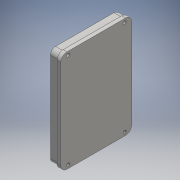
# Autodesk Inventor part: ET7
Saved by Autodesk Inventor 2016 (Build 200138000, 138)
## iProperties
Created: 2016-03-20
Part Number: ET7
Material: Genérico
Document SubType Name: Modeling
Designer: Usuario1
Density: 1 g/cm^3
Appearance: Valor por defecto
Author: Usuario1
Autodesk Inventor part; units mm, degrees
ref_plane "YZ Plane" through (0, 0, 0) normal (1, 0, 0) x (0, 1, 0)
ref_plane "XZ Plane" through (0, 0, 0) normal (0, 1, 0) x (-1, 0, 0)
ref_plane "XY Plane" through (0, 0, 0) normal (0, 0, 1) x (1, 0, 0)
sketch "Boceto1" plane through (0, 0, 0) normal (1, 0, 0) x (0, 1, 0)
  line L0 (2.3957, 0.3049) -> (2.3957, 0.0787)
  line L1 (2.3957, 0.0787) -> (2.2436, 0.0787)
  line L2 (2.2436, 0.0787) -> (2.2436, 0.3049)
  line L3 (2.2436, 0.3049) -> (2.3957, 0.3049)
  circle A0 centre (0.5248, 3.3826) radius 0.0547
  line L4 (0.5812, 3.113) -> (0.5812, 2.8452)
  line L5 (0.5812, 2.8452) -> (0.4683, 2.8452)
  line L6 (0.4683, 2.8452) -> (0.4683, 3.113)
  line L7 (0.4683, 3.113) -> (0.5812, 3.113)
  line L8 (0.5812, 2.5971) -> (0.5812, 2.3293)
  line L9 (0.5812, 2.3293) -> (0.4683, 2.3293)
  line L10 (0.4683, 2.3293) -> (0.4683, 2.5971)
  line L11 (0.4683, 2.5971) -> (0.5812, 2.5971)
  line L12 (0.5812, 2.0812) -> (0.5812, 1.8134)
  line L13 (0.5812, 1.8134) -> (0.4683, 1.8134)
  line L14 (0.4683, 1.8134) -> (0.4683, 2.0812)
  line L15 (0.4683, 2.0812) -> (0.5812, 2.0812)
  line L16 (0.5812, 1.5653) -> (0.5812, 1.2975)
  line L17 (0.5812, 1.2975) -> (0.4683, 1.2975)
  line L18 (0.4683, 1.2975) -> (0.4683, 1.5653)
  line L19 (0.4683, 1.5653) -> (0.5812, 1.5653)
  line L20 (0.5812, 1.0494) -> (0.5812, 0.7816)
  line L21 (0.5812, 0.7816) -> (0.4683, 0.7816)
  line L22 (0.4683, 0.7816) -> (0.4683, 1.0494)
  line L23 (0.4683, 1.0494) -> (0.5812, 1.0494)
  line L24 (1.2433, 0.3049) -> (1.2433, 0.0787)
  line L25 (1.2433, 0.0787) -> (1.0912, 0.0787)
  line L26 (1.0912, 0.0787) -> (1.0912, 0.3049)
  line L27 (1.0912, 0.3049) -> (1.2433, 0.3049)
  line L28 (0.5861, 0.3049) -> (0.5861, 0.0787)
  line L29 (0.5861, 0.0787) -> (0.434, 0.0787)
  line L30 (0.434, 0.0787) -> (0.434, 0.3049)
  line L31 (0.434, 0.3049) -> (0.5861, 0.3049)
  line L32 (2.7629, 3.0481) -> (2.7629, 2.6834)
  line L33 (2.7629, 2.6834) -> (2.9608, 2.6834)
  line L34 (2.9608, 2.6834) -> (2.9608, 3.0481)
  line L35 (2.9608, 3.0481) -> (2.7629, 3.0481)
  line L36 (2.7629, 2.4411) -> (2.7629, 1.0453)
  line L37 (2.7629, 1.0453) -> (2.817, 1.0453)
  line L38 (2.817, 1.0453) -> (2.817, 2.4411)
  line L39 (2.817, 2.4411) -> (2.7629, 2.4411)
  circle A1 centre (2.483, -0.1054) radius 0.0623
  circle A2 centre (0.2799, -0.1054) radius 0.0623
  circle A3 centre (0.2799, 3.5918) radius 0.0623
  line L40 (2.7629, 3.4863) -> (2.7629, 0)
  arc A4 (2.5229, -0.24) -> (2.7629, 0) centre (2.5229, 0) ccw
  line L41 (2.5229, -0.24) -> (0.24, -0.24)
  arc A5 (0, 0) -> (0.24, -0.24) centre (0.24, 0) ccw
  line L42 (0, 0) -> (0, 3.4863)
  arc A6 (0.24, 3.7263) -> (0, 3.4863) centre (0.24, 3.4863) ccw
  line L43 (0.24, 3.7263) -> (2.5229, 3.7263)
  arc A7 (2.7629, 3.4863) -> (2.5229, 3.7263) centre (2.5229, 3.4863) ccw
  line L44 (0.0443, 3.4821) -> (0.0443, 0.0043)
  arc A8 (0.0443, 0.0043) -> (0.2443, -0.1957) centre (0.2443, 0.0043) ccw
  line L45 (0.2443, -0.1957) -> (2.5186, -0.1957)
  arc A9 (2.5186, -0.1957) -> (2.7186, 0.0043) centre (2.5186, 0.0043) ccw
  line L46 (2.7186, 0.0043) -> (2.7186, 3.4821)
  arc A10 (2.7186, 3.4821) -> (2.5186, 3.6821) centre (2.5186, 3.4821) ccw
  line L47 (2.5186, 3.6821) -> (0.2443, 3.6821)
  arc A11 (0.2443, 3.6821) -> (0.0443, 3.4821) centre (0.2443, 3.4821) ccw
  circle A12 centre (2.483, 3.5918) radius 0.0623
  line L48 (2.5087, 3.3303) -> (2.5087, 0.538)
  arc A13 (2.3887, 0.418) -> (2.5087, 0.538) centre (2.3887, 0.538) ccw
  line L49 (2.3887, 0.418) -> (0.8107, 0.418)
  arc A14 (0.6907, 0.538) -> (0.8107, 0.418) centre (0.8107, 0.538) ccw
  line L50 (0.6907, 0.538) -> (0.6907, 3.3303)
  arc A15 (0.8107, 3.4503) -> (0.6907, 3.3303) centre (0.8107, 3.3303) ccw
  line L51 (0.8107, 3.4503) -> (2.3887, 3.4503)
  arc A16 (2.5087, 3.3303) -> (2.3887, 3.4503) centre (2.3887, 3.3303) ccw
  line L52 (2.4044, 3.2168) -> (2.4044, 0.6515)
  arc A17 (2.3144, 0.5615) -> (2.4044, 0.6515) centre (2.3144, 0.6515) ccw
  line L53 (2.3144, 0.5615) -> (0.9806, 0.5615)
  arc A18 (0.8906, 0.6515) -> (0.9806, 0.5615) centre (0.9806, 0.6515) ccw
  line L54 (0.8906, 0.6515) -> (0.8906, 3.2168)
  arc A19 (0.9806, 3.3068) -> (0.8906, 3.2168) centre (0.9806, 3.2168) ccw
  line L55 (0.9806, 3.3068) -> (2.3144, 3.3068)
  arc A20 (2.4044, 3.2168) -> (2.3144, 3.3068) centre (2.3144, 3.2168) ccw
  point P0 (0, 0)
  constraints: 112 end point, 32 point on circle, 21 centre point, 4 point on line
extrude "Extrusión1" add sketch "Boceto1" against normal blind 0.15 contours L0 L1 L2 L3 | A0 | L4 L5 L6 L7 | L8 L9 L10 L11 | L12 L13 L14 L15 | L16 L17 L18 L19 | L20 L21 L22 L23 | L24 L25 L26 L27 | L28 L29 L30 L31 | L32 L40 L36 A4 L41 A5 L42 A6 L43 A7 | A11 L47 A10 L46 A9 L45 A8 L44 | L48 A13 L49 A14 L50 A15 L51 A16 | L52 A17 L53 A18 L54 A19 L55 A20
sketch "Boceto2" plane through (-0.15, 0, 0) normal (-1, 0, 0) x (0, 0, 1)
  circle A0 centre (3.5918, 2.483) radius 0.0623 projected
  circle A1 centre (3.5918, 0.2799) radius 0.0623 projected
  circle A2 centre (-0.1054, 0.2799) radius 0.0623 projected
  circle A3 centre (-0.1054, 2.483) radius 0.0623 projected
  line L0 (3.1814, 2.3957) -> (3.4077, 2.3957)
  line L1 (3.4077, 2.3957) -> (3.4077, 2.2436)
  line L2 (3.4077, 2.2436) -> (3.1814, 2.2436)
  line L3 (3.1814, 2.2436) -> (3.1814, 2.3957)
  circle A4 centre (0.1037, 0.5248) radius 0.0547
  line L4 (0.3734, 0.5812) -> (0.6411, 0.5812)
  line L5 (0.6411, 0.5812) -> (0.6411, 0.4683)
  line L6 (0.6411, 0.4683) -> (0.3734, 0.4683)
  line L7 (0.3734, 0.4683) -> (0.3734, 0.5812)
  line L8 (0.8893, 0.5812) -> (1.157, 0.5812)
  line L9 (1.157, 0.5812) -> (1.157, 0.4683)
  line L10 (1.157, 0.4683) -> (0.8893, 0.4683)
  line L11 (0.8893, 0.4683) -> (0.8893, 0.5812)
  line L12 (1.4052, 0.5812) -> (1.6729, 0.5812)
  line L13 (1.6729, 0.5812) -> (1.6729, 0.4683)
  line L14 (1.6729, 0.4683) -> (1.4052, 0.4683)
  line L15 (1.4052, 0.4683) -> (1.4052, 0.5812)
  line L16 (1.921, 0.5812) -> (2.1888, 0.5812)
  line L17 (2.1888, 0.5812) -> (2.1888, 0.4683)
  line L18 (2.1888, 0.4683) -> (1.921, 0.4683)
  line L19 (1.921, 0.4683) -> (1.921, 0.5812)
  line L20 (2.4369, 0.5812) -> (2.7047, 0.5812)
  line L21 (2.7047, 0.5812) -> (2.7047, 0.4683)
  line L22 (2.7047, 0.4683) -> (2.4369, 0.4683)
  line L23 (2.4369, 0.4683) -> (2.4369, 0.5812)
  line L24 (3.1814, 1.2433) -> (3.4077, 1.2433)
  line L25 (3.4077, 1.2433) -> (3.4077, 1.0912)
  line L26 (3.4077, 1.0912) -> (3.1814, 1.0912)
  line L27 (3.1814, 1.0912) -> (3.1814, 1.2433)
  line L28 (3.1814, 0.5861) -> (3.4077, 0.5861)
  line L29 (3.4077, 0.5861) -> (3.4077, 0.434)
  line L30 (3.4077, 0.434) -> (3.1814, 0.434)
  line L31 (3.1814, 0.434) -> (3.1814, 0.5861)
  line L32 (0.4382, 2.7629) -> (0.803, 2.7629)
  line L33 (0.803, 2.7629) -> (0.803, 2.9608)
  line L34 (0.803, 2.9608) -> (0.4382, 2.9608)
  line L35 (0.4382, 2.9608) -> (0.4382, 2.7629)
  line L36 (1.0453, 2.7629) -> (2.4411, 2.7629)
  line L37 (2.4411, 2.7629) -> (2.4411, 2.817)
  line L38 (2.4411, 2.817) -> (1.0453, 2.817)
  line L39 (1.0453, 2.817) -> (1.0453, 2.7629)
  circle A5 centre (3.5918, 2.483) radius 0.0623
  circle A6 centre (3.5918, 0.2799) radius 0.0623
  circle A7 centre (-0.1054, 0.2799) radius 0.0623
  line L40 (0, 2.7629) -> (3.4863, 2.7629)
  arc A8 (3.7263, 2.5229) -> (3.4863, 2.7629) centre (3.4863, 2.5229) ccw
  line L41 (3.7263, 2.5229) -> (3.7263, 0.24)
  arc A9 (3.4863, 0) -> (3.7263, 0.24) centre (3.4863, 0.24) ccw
  line L42 (3.4863, 0) -> (0, 0)
  arc A10 (-0.24, 0.24) -> (0, 0) centre (0, 0.24) ccw
  line L43 (-0.24, 0.24) -> (-0.24, 2.5229)
  arc A11 (0, 2.7629) -> (-0.24, 2.5229) centre (0, 2.5229) ccw
  line L44 (0.0043, 0.0443) -> (3.4821, 0.0443)
  arc A12 (3.4821, 0.0443) -> (3.6821, 0.2443) centre (3.4821, 0.2443) ccw
  line L45 (3.6821, 0.2443) -> (3.6821, 2.5186)
  arc A13 (3.6821, 2.5186) -> (3.4821, 2.7186) centre (3.4821, 2.5186) ccw
  line L46 (3.4821, 2.7186) -> (0.0043, 2.7186)
  arc A14 (0.0043, 2.7186) -> (-0.1957, 2.5186) centre (0.0043, 2.5186) ccw
  line L47 (-0.1957, 2.5186) -> (-0.1957, 0.2443)
  arc A15 (-0.1957, 0.2443) -> (0.0043, 0.0443) centre (0.0043, 0.2443) ccw
  circle A16 centre (-0.1054, 2.483) radius 0.0623
  line L48 (0.1561, 2.5087) -> (2.9483, 2.5087)
  arc A17 (3.0683, 2.3887) -> (2.9483, 2.5087) centre (2.9483, 2.3887) ccw
  line L49 (3.0683, 2.3887) -> (3.0683, 0.8107)
  arc A18 (2.9483, 0.6907) -> (3.0683, 0.8107) centre (2.9483, 0.8107) ccw
  line L50 (2.9483, 0.6907) -> (0.1561, 0.6907)
  arc A19 (0.0361, 0.8107) -> (0.1561, 0.6907) centre (0.1561, 0.8107) ccw
  line L51 (0.0361, 0.8107) -> (0.0361, 2.3887)
  arc A20 (0.1561, 2.5087) -> (0.0361, 2.3887) centre (0.1561, 2.3887) ccw
  line L52 (0.2695, 2.4044) -> (2.8349, 2.4044)
  arc A21 (2.9249, 2.3144) -> (2.8349, 2.4044) centre (2.8349, 2.3144) ccw
  line L53 (2.9249, 2.3144) -> (2.9249, 0.9806)
  arc A22 (2.8349, 0.8906) -> (2.9249, 0.9806) centre (2.8349, 0.9806) ccw
  line L54 (2.8349, 0.8906) -> (0.2695, 0.8906)
  arc A23 (0.1795, 0.9806) -> (0.2695, 0.8906) centre (0.2695, 0.9806) ccw
  line L55 (0.1795, 0.9806) -> (0.1795, 2.3144)
  arc A24 (0.2695, 2.4044) -> (0.1795, 2.3144) centre (0.2695, 2.3144) ccw
  point P0 (0, 0)
  constraints: 112 end point, 32 point on circle, 21 centre point, 4 point on line
extrude "Extrusión2" add sketch "Boceto2" along normal blind 0.3 contours L0 L1 L2 L3 | A4 | L4 L5 L6 L7 | L8 L9 L10 L11 | L12 L13 L14 L15 | L16 L17 L18 L19 | L20 L21 L22 L23 | L24 L25 L26 L27 | L28 L29 L30 L31 | A15 L47 A14 L46 A13 L45 A12 L44 | L48 A17 L49 A18 L50 A19 L51 A20 | L52 A21 L53 A22 L54 A23 L55 A24
sketch "Boceto3" plane through (-0.45, 0, 0) normal (-1, 0, 0) x (0, 0, 1)
  circle A0 centre (-0.1054, 2.483) radius 0.0623 projected
  circle A1 centre (-0.1054, 0.2799) radius 0.0623 projected
  circle A2 centre (3.5918, 0.2799) radius 0.0623 projected
  circle A3 centre (3.5918, 2.483) radius 0.0623 projected
  line L0 (0.0043, 0.0443) -> (3.4821, 0.0443) projected
  arc A4 (3.4821, 0.0443) -> (3.6821, 0.2443) centre (3.4821, 0.2443) ccw projected
  line L1 (3.6821, 0.2443) -> (3.6821, 2.5186) projected
  arc A5 (3.6821, 2.5186) -> (3.4821, 2.7186) centre (3.4821, 2.5186) ccw projected
  line L2 (3.4821, 2.7186) -> (0.0043, 2.7186) projected
  arc A6 (0.0043, 2.7186) -> (-0.1957, 2.5186) centre (0.0043, 2.5186) ccw projected
  line L3 (-0.1957, 2.5186) -> (-0.1957, 0.2443) projected
  arc A7 (-0.1957, 0.2443) -> (0.0043, 0.0443) centre (0.0043, 0.2443) ccw projected
  line L4 (3.1814, 2.3957) -> (3.4077, 2.3957)
  line L5 (3.4077, 2.3957) -> (3.4077, 2.2436)
  line L6 (3.4077, 2.2436) -> (3.1814, 2.2436)
  line L7 (3.1814, 2.2436) -> (3.1814, 2.3957)
  circle A8 centre (0.1037, 0.5248) radius 0.0547
  line L8 (0.3734, 0.5812) -> (0.6411, 0.5812)
  line L9 (0.6411, 0.5812) -> (0.6411, 0.4683)
  line L10 (0.6411, 0.4683) -> (0.3734, 0.4683)
  line L11 (0.3734, 0.4683) -> (0.3734, 0.5812)
  line L12 (0.8893, 0.5812) -> (1.157, 0.5812)
  line L13 (1.157, 0.5812) -> (1.157, 0.4683)
  line L14 (1.157, 0.4683) -> (0.8893, 0.4683)
  line L15 (0.8893, 0.4683) -> (0.8893, 0.5812)
  line L16 (1.4052, 0.5812) -> (1.6729, 0.5812)
  line L17 (1.6729, 0.5812) -> (1.6729, 0.4683)
  line L18 (1.6729, 0.4683) -> (1.4052, 0.4683)
  line L19 (1.4052, 0.4683) -> (1.4052, 0.5812)
  line L20 (1.921, 0.5812) -> (2.1888, 0.5812)
  line L21 (2.1888, 0.5812) -> (2.1888, 0.4683)
  line L22 (2.1888, 0.4683) -> (1.921, 0.4683)
  line L23 (1.921, 0.4683) -> (1.921, 0.5812)
  line L24 (2.4369, 0.5812) -> (2.7047, 0.5812)
  line L25 (2.7047, 0.5812) -> (2.7047, 0.4683)
  line L26 (2.7047, 0.4683) -> (2.4369, 0.4683)
  line L27 (2.4369, 0.4683) -> (2.4369, 0.5812)
  line L28 (3.1814, 1.2433) -> (3.4077, 1.2433)
  line L29 (3.4077, 1.2433) -> (3.4077, 1.0912)
  line L30 (3.4077, 1.0912) -> (3.1814, 1.0912)
  line L31 (3.1814, 1.0912) -> (3.1814, 1.2433)
  line L32 (3.1814, 0.5861) -> (3.4077, 0.5861)
  line L33 (3.4077, 0.5861) -> (3.4077, 0.434)
  line L34 (3.4077, 0.434) -> (3.1814, 0.434)
  line L35 (3.1814, 0.434) -> (3.1814, 0.5861)
  line L36 (0.4382, 2.7629) -> (0.803, 2.7629)
  line L37 (0.803, 2.7629) -> (0.803, 2.9608)
  line L38 (0.803, 2.9608) -> (0.4382, 2.9608)
  line L39 (0.4382, 2.9608) -> (0.4382, 2.7629)
  line L40 (1.0453, 2.7629) -> (2.4411, 2.7629)
  line L41 (2.4411, 2.7629) -> (2.4411, 2.817)
  line L42 (2.4411, 2.817) -> (1.0453, 2.817)
  line L43 (1.0453, 2.817) -> (1.0453, 2.7629)
  circle A9 centre (3.5918, 2.483) radius 0.0623
  circle A10 centre (3.5918, 0.2799) radius 0.0623
  circle A11 centre (-0.1054, 0.2799) radius 0.0623
  line L44 (0, 2.7629) -> (3.4863, 2.7629)
  arc A12 (3.7263, 2.5229) -> (3.4863, 2.7629) centre (3.4863, 2.5229) ccw
  line L45 (3.7263, 2.5229) -> (3.7263, 0.24)
  arc A13 (3.4863, 0) -> (3.7263, 0.24) centre (3.4863, 0.24) ccw
  line L46 (3.4863, 0) -> (0, 0)
  arc A14 (-0.24, 0.24) -> (0, 0) centre (0, 0.24) ccw
  line L47 (-0.24, 0.24) -> (-0.24, 2.5229)
  arc A15 (0, 2.7629) -> (-0.24, 2.5229) centre (0, 2.5229) ccw
  line L48 (0.0043, 0.0443) -> (3.4821, 0.0443)
  arc A16 (3.4821, 0.0443) -> (3.6821, 0.2443) centre (3.4821, 0.2443) ccw
  line L49 (3.6821, 0.2443) -> (3.6821, 2.5186)
  arc A17 (3.6821, 2.5186) -> (3.4821, 2.7186) centre (3.4821, 2.5186) ccw
  line L50 (3.4821, 2.7186) -> (0.0043, 2.7186)
  arc A18 (0.0043, 2.7186) -> (-0.1957, 2.5186) centre (0.0043, 2.5186) ccw
  line L51 (-0.1957, 2.5186) -> (-0.1957, 0.2443)
  arc A19 (-0.1957, 0.2443) -> (0.0043, 0.0443) centre (0.0043, 0.2443) ccw
  circle A20 centre (-0.1054, 2.483) radius 0.0623
  line L52 (0.1561, 2.5087) -> (2.9483, 2.5087)
  arc A21 (3.0683, 2.3887) -> (2.9483, 2.5087) centre (2.9483, 2.3887) ccw
  line L53 (3.0683, 2.3887) -> (3.0683, 0.8107)
  arc A22 (2.9483, 0.6907) -> (3.0683, 0.8107) centre (2.9483, 0.8107) ccw
  line L54 (2.9483, 0.6907) -> (0.1561, 0.6907)
  arc A23 (0.0361, 0.8107) -> (0.1561, 0.6907) centre (0.1561, 0.8107) ccw
  line L55 (0.0361, 0.8107) -> (0.0361, 2.3887)
  arc A24 (0.1561, 2.5087) -> (0.0361, 2.3887) centre (0.1561, 2.3887) ccw
  line L56 (0.2695, 2.4044) -> (2.8349, 2.4044)
  arc A25 (2.9249, 2.3144) -> (2.8349, 2.4044) centre (2.8349, 2.3144) ccw
  line L57 (2.9249, 2.3144) -> (2.9249, 0.9806)
  arc A26 (2.8349, 0.8906) -> (2.9249, 0.9806) centre (2.8349, 0.9806) ccw
  line L58 (2.8349, 0.8906) -> (0.2695, 0.8906)
  arc A27 (0.1795, 0.9806) -> (0.2695, 0.8906) centre (0.2695, 0.9806) ccw
  line L59 (0.1795, 0.9806) -> (0.1795, 2.3144)
  arc A28 (0.2695, 2.4044) -> (0.1795, 2.3144) centre (0.2695, 2.3144) ccw
  point P0 (0, 0)
  constraints: 112 end point, 32 point on circle, 21 centre point, 4 point on line
extrude "Extrusión3" add sketch "Boceto3" along normal blind 0.04 contours L4 L5 L6 L7 | A8 | L8 L9 L10 L11 | L12 L13 L14 L15 | L16 L17 L18 L19 | L20 L21 L22 L23 | L24 L25 L26 L27 | L28 L29 L30 L31 | L32 L33 L34 L35
sketch "Boceto4" plane through (-0.45, 0, 0) normal (-1, 0, 0) x (0, 0, 1)
  line L0 (3.4077, 1.2433) -> (3.4077, 1.0912) projected
  line L1 (3.4077, 1.0912) -> (3.1814, 1.0912) projected
  line L2 (3.1814, 1.0912) -> (3.1814, 1.2433) projected
  line L3 (3.1814, 1.2433) -> (3.4077, 1.2433) projected
  line L4 (2.7047, 0.5812) -> (2.7047, 0.4683) projected
  line L5 (2.7047, 0.4683) -> (2.4369, 0.4683) projected
  line L6 (2.4369, 0.4683) -> (2.4369, 0.5812) projected
  line L7 (2.4369, 0.5812) -> (2.7047, 0.5812) projected
  line L8 (1.6729, 0.5812) -> (1.6729, 0.4683) projected
  line L9 (1.6729, 0.4683) -> (1.4052, 0.4683) projected
  line L10 (1.4052, 0.4683) -> (1.4052, 0.5812) projected
  line L11 (1.4052, 0.5812) -> (1.6729, 0.5812) projected
  line L12 (0.6411, 0.5812) -> (0.6411, 0.4683) projected
  line L13 (0.6411, 0.4683) -> (0.3734, 0.4683) projected
  line L14 (0.3734, 0.4683) -> (0.3734, 0.5812) projected
  line L15 (0.3734, 0.5812) -> (0.6411, 0.5812) projected
  circle A0 centre (0.1037, 0.5248) radius 0.0547 projected
  line L16 (1.157, 0.5812) -> (1.157, 0.4683) projected
  line L17 (1.157, 0.4683) -> (0.8893, 0.4683) projected
  line L18 (0.8893, 0.4683) -> (0.8893, 0.5812) projected
  line L19 (0.8893, 0.5812) -> (1.157, 0.5812) projected
  line L20 (2.1888, 0.5812) -> (2.1888, 0.4683) projected
  line L21 (2.1888, 0.4683) -> (1.921, 0.4683) projected
  line L22 (1.921, 0.4683) -> (1.921, 0.5812) projected
  line L23 (1.921, 0.5812) -> (2.1888, 0.5812) projected
  line L24 (3.4077, 2.3957) -> (3.4077, 2.2436) projected
  line L25 (3.4077, 2.2436) -> (3.1814, 2.2436) projected
  line L26 (3.1814, 2.2436) -> (3.1814, 2.3957) projected
  line L27 (3.1814, 2.3957) -> (3.4077, 2.3957) projected
  line L28 (3.4077, 0.5861) -> (3.4077, 0.434) projected
  line L29 (3.4077, 0.434) -> (3.1814, 0.434) projected
  line L30 (3.1814, 0.434) -> (3.1814, 0.5861) projected
  line L31 (3.1814, 0.5861) -> (3.4077, 0.5861) projected
  circle A1 centre (-0.1054, 2.483) radius 0.0623 projected
  circle A2 centre (-0.1054, 0.2799) radius 0.0623 projected
  circle A3 centre (3.5918, 0.2799) radius 0.0623 projected
  circle A4 centre (3.5918, 2.483) radius 0.0623 projected
  line L32 (0.0043, 0.0443) -> (3.4821, 0.0443) projected
  arc A5 (3.4821, 0.0443) -> (3.6821, 0.2443) centre (3.4821, 0.2443) ccw projected
  line L33 (3.6821, 0.2443) -> (3.6821, 2.5186) projected
  arc A6 (3.6821, 2.5186) -> (3.4821, 2.7186) centre (3.4821, 2.5186) ccw projected
  line L34 (3.4821, 2.7186) -> (0.0043, 2.7186) projected
  arc A7 (0.0043, 2.7186) -> (-0.1957, 2.5186) centre (0.0043, 2.5186) ccw projected
  line L35 (-0.1957, 2.5186) -> (-0.1957, 0.2443) projected
  arc A8 (-0.1957, 0.2443) -> (0.0043, 0.0443) centre (0.0043, 0.2443) ccw projected
  line L36 (3.1814, 2.3957) -> (3.4077, 2.3957)
  line L37 (3.4077, 2.3957) -> (3.4077, 2.2436)
  line L38 (3.4077, 2.2436) -> (3.1814, 2.2436)
  line L39 (3.1814, 2.2436) -> (3.1814, 2.3957)
  circle A9 centre (0.1037, 0.5248) radius 0.0547
  line L40 (0.3734, 0.5812) -> (0.6411, 0.5812)
  line L41 (0.6411, 0.5812) -> (0.6411, 0.4683)
  line L42 (0.6411, 0.4683) -> (0.3734, 0.4683)
  line L43 (0.3734, 0.4683) -> (0.3734, 0.5812)
  line L44 (0.8893, 0.5812) -> (1.157, 0.5812)
  line L45 (1.157, 0.5812) -> (1.157, 0.4683)
  line L46 (1.157, 0.4683) -> (0.8893, 0.4683)
  line L47 (0.8893, 0.4683) -> (0.8893, 0.5812)
  line L48 (1.4052, 0.5812) -> (1.6729, 0.5812)
  line L49 (1.6729, 0.5812) -> (1.6729, 0.4683)
  line L50 (1.6729, 0.4683) -> (1.4052, 0.4683)
  line L51 (1.4052, 0.4683) -> (1.4052, 0.5812)
  line L52 (1.921, 0.5812) -> (2.1888, 0.5812)
  line L53 (2.1888, 0.5812) -> (2.1888, 0.4683)
  line L54 (2.1888, 0.4683) -> (1.921, 0.4683)
  line L55 (1.921, 0.4683) -> (1.921, 0.5812)
  line L56 (2.4369, 0.5812) -> (2.7047, 0.5812)
  line L57 (2.7047, 0.5812) -> (2.7047, 0.4683)
  line L58 (2.7047, 0.4683) -> (2.4369, 0.4683)
  line L59 (2.4369, 0.4683) -> (2.4369, 0.5812)
  line L60 (3.1814, 1.2433) -> (3.4077, 1.2433)
  line L61 (3.4077, 1.2433) -> (3.4077, 1.0912)
  line L62 (3.4077, 1.0912) -> (3.1814, 1.0912)
  line L63 (3.1814, 1.0912) -> (3.1814, 1.2433)
  line L64 (3.1814, 0.5861) -> (3.4077, 0.5861)
  line L65 (3.4077, 0.5861) -> (3.4077, 0.434)
  line L66 (3.4077, 0.434) -> (3.1814, 0.434)
  line L67 (3.1814, 0.434) -> (3.1814, 0.5861)
  line L68 (0.4382, 2.7629) -> (0.803, 2.7629)
  line L69 (0.803, 2.7629) -> (0.803, 2.9608)
  line L70 (0.803, 2.9608) -> (0.4382, 2.9608)
  line L71 (0.4382, 2.9608) -> (0.4382, 2.7629)
  line L72 (1.0453, 2.7629) -> (2.4411, 2.7629)
  line L73 (2.4411, 2.7629) -> (2.4411, 2.817)
  line L74 (2.4411, 2.817) -> (1.0453, 2.817)
  line L75 (1.0453, 2.817) -> (1.0453, 2.7629)
  circle A10 centre (3.5918, 2.483) radius 0.0623
  circle A11 centre (3.5918, 0.2799) radius 0.0623
  circle A12 centre (-0.1054, 0.2799) radius 0.0623
  line L76 (0, 2.7629) -> (3.4863, 2.7629)
  arc A13 (3.7263, 2.5229) -> (3.4863, 2.7629) centre (3.4863, 2.5229) ccw
  line L77 (3.7263, 2.5229) -> (3.7263, 0.24)
  arc A14 (3.4863, 0) -> (3.7263, 0.24) centre (3.4863, 0.24) ccw
  line L78 (3.4863, 0) -> (0, 0)
  arc A15 (-0.24, 0.24) -> (0, 0) centre (0, 0.24) ccw
  line L79 (-0.24, 0.24) -> (-0.24, 2.5229)
  arc A16 (0, 2.7629) -> (-0.24, 2.5229) centre (0, 2.5229) ccw
  line L80 (0.0043, 0.0443) -> (3.4821, 0.0443)
  arc A17 (3.4821, 0.0443) -> (3.6821, 0.2443) centre (3.4821, 0.2443) ccw
  line L81 (3.6821, 0.2443) -> (3.6821, 2.5186)
  arc A18 (3.6821, 2.5186) -> (3.4821, 2.7186) centre (3.4821, 2.5186) ccw
  line L82 (3.4821, 2.7186) -> (0.0043, 2.7186)
  arc A19 (0.0043, 2.7186) -> (-0.1957, 2.5186) centre (0.0043, 2.5186) ccw
  line L83 (-0.1957, 2.5186) -> (-0.1957, 0.2443)
  arc A20 (-0.1957, 0.2443) -> (0.0043, 0.0443) centre (0.0043, 0.2443) ccw
  circle A21 centre (-0.1054, 2.483) radius 0.0623
  line L84 (0.1561, 2.5087) -> (2.9483, 2.5087)
  arc A22 (3.0683, 2.3887) -> (2.9483, 2.5087) centre (2.9483, 2.3887) ccw
  line L85 (3.0683, 2.3887) -> (3.0683, 0.8107)
  arc A23 (2.9483, 0.6907) -> (3.0683, 0.8107) centre (2.9483, 0.8107) ccw
  line L86 (2.9483, 0.6907) -> (0.1561, 0.6907)
  arc A24 (0.0361, 0.8107) -> (0.1561, 0.6907) centre (0.1561, 0.8107) ccw
  line L87 (0.0361, 0.8107) -> (0.0361, 2.3887)
  arc A25 (0.1561, 2.5087) -> (0.0361, 2.3887) centre (0.1561, 2.3887) ccw
  line L88 (0.2695, 2.4044) -> (2.8349, 2.4044)
  arc A26 (2.9249, 2.3144) -> (2.8349, 2.4044) centre (2.8349, 2.3144) ccw
  line L89 (2.9249, 2.3144) -> (2.9249, 0.9806)
  arc A27 (2.8349, 0.8906) -> (2.9249, 0.9806) centre (2.8349, 0.9806) ccw
  line L90 (2.8349, 0.8906) -> (0.2695, 0.8906)
  arc A28 (0.1795, 0.9806) -> (0.2695, 0.8906) centre (0.2695, 0.9806) ccw
  line L91 (0.1795, 0.9806) -> (0.1795, 2.3144)
  arc A29 (0.2695, 2.4044) -> (0.1795, 2.3144) centre (0.2695, 2.3144) ccw
  point P0 (0, 0)
  constraints: 112 end point, 32 point on circle, 21 centre point, 4 point on line
extrude "Extrusión4" add sketch "Boceto4" along normal blind 0.02 contours L84 A22 L85 A23 L86 A24 L87 A25
